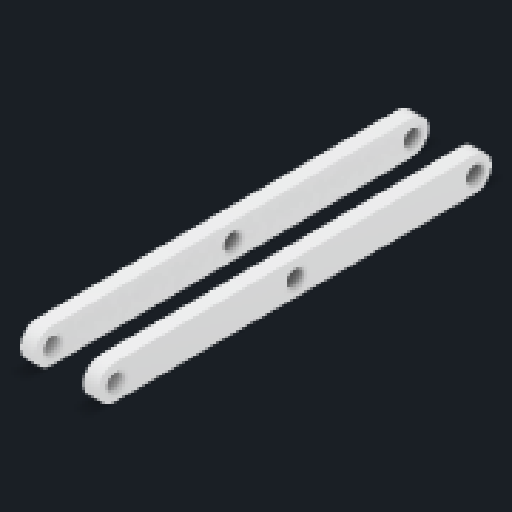
# Autodesk Inventor part: Corredera I
Saved by Autodesk Inventor 2025.3 (Build 293356030, 356C)
## iProperties
Created: 2024-11-12
Part Number: Corredera I
Material: Aluminio 6061
Document SubType Name: Modeling
Designer: j.santaa
Density: 2.7 g/cm^3
Appearance: Aluminio - Plano
Mass: 3.54373 g
Surface Area: 36.8835 cm^2
Volume: 3.54373 cm^3
Author: j.santaa
Autodesk Inventor part; units mm, degrees
ref_plane "YZ Plane" through (0, 0, 0) normal (1, 0, 0) x (0, 1, 0)
ref_plane "XZ Plane" through (0, 0, 0) normal (0, 1, 0) x (-1, 0, 0)
ref_plane "XY Plane" through (0, 0, 0) normal (0, 0, 1) x (1, 0, 0)
sketch "Sketch1" plane through (0, 0, 0) normal (1, 0, 0) x (0, 1, 0)
  line L0 (0, 37) -> (0, -37) construction
  line L1 (-3.5, 37) -> (-3.5, -37)
  line L2 (3.5, -37) -> (3.5, 37)
  arc A0 (3.5, 37) -> (-3.5, 37) centre (0, 37) ccw
  arc A1 (-3.5, -37) -> (3.5, -37) centre (0, -37) ccw
  circle A2 centre (0, -37) radius 1.5
  circle A3 centre (0, 0) radius 1.5
  circle A4 centre (0, 37) radius 1.5
  point P0 (0, 40.5)
  point P1 (0, -40.5)
  dimension "d14" = 7
  dimension "d15" = 81
  dimension "d16" = 3
  constraints: 8 end point, 6 point on circle, 5 centre point, 4 coincident, 4 tangent, 2 equal radius, 1 midpoint, 1 parallel, 1 vertical
  measures "d14" diameter of A1
  measures "d15" distance of point (0, 40.5) point (0, -40.5)
  measures "d16" diameter of A2
extrude "Extrusión3" add sketch "Sketch1" along normal mid plane 16 contours A0 L2 A1 L1 | A2 | A3 | A4
extrude "Extrusión4" cut sketch "Sketch1" along normal mid plane 10 contours A0 L2 A1 L1 | A3
sketch "Boceto2" plane through (-8, 0, 0) normal (-1, 0, 0) x (0, 0, 1)
  circle A0 centre (37, 0) radius 1.5 projected
  circle A1 centre (-37, 0) radius 1.5 projected
  point P0 (0, 0)
  point P1 (0, 0)
  constraints: 3 coincident
hole "Agujero1" at (-8, 0, 37) at (-8, 0, -37) at (-8, 0, 0) direction (1, 0, 0) diameter 3.4 end through all clearance for "Tornillo de cabeza plana avellanada ISO 2009/7046" size "M3" standard "ISO"
equation "\"d19\" = Dedos"
equation "\"Dedos\" = 10"
